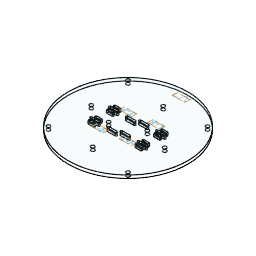
TopPlate_v24 (Autodesk Fusion 360 design; units mm, degrees)
Autodesk Fusion 360 part; units mm, degrees
sketch "Sketch1" plane through (0, 0, 0) normal (0, 0, 1) x (1, 0, 0)
  circle A0 centre (0, 0) radius 59.5
  line L0 (0, -35) -> (0, 35) construction
  circle A1 centre (0, -35) radius 1.75
  circle A2 centre (0, 35) radius 3
  circle A3 centre (0, -35) radius 3
  circle A4 centre (0, 35) radius 6
  circle A5 centre (0, -35) radius 6
  circle A6 centre (0, 35) radius 1.75
  line L1 (0, 0) -> (39.598, 39.598) construction
  line L2 (0, 0) -> (53.8605, 0) construction
  circle A7 centre (39.598, 39.598) radius 1.75
  circle A8 centre (-39.598, 39.598) radius 1.75
  circle A9 centre (-39.598, -39.598) radius 1.75
  circle A10 centre (39.598, -39.598) radius 1.75
  line L3 (-26, 7.75) -> (-1, 7.75) construction
  circle A11 centre (-26, 7.75) radius 1
  circle A12 centre (-1, 7.75) radius 1
  circle A13 centre (-18, 7.75) radius 1
  circle A14 centre (-9, 7.75) radius 1
  line L4 (-26, 8.75) -> (-18, 8.75)
  line L5 (-18, 6.75) -> (-26, 6.75)
  line L6 (-9, 8.75) -> (-1, 8.75)
  line L7 (-1, 6.75) -> (-9, 6.75)
  line L8 (0, 0) -> (-1, 0)
  line L9 (-1, 0) -> (-1, 7.75) construction
  line L10 (26, -8.75) -> (18, -8.75)
  circle A15 centre (26, -7.75) radius 1
  line L11 (18, -6.75) -> (26, -6.75)
  circle A16 centre (18, -7.75) radius 1
  circle A17 centre (9, -7.75) radius 1
  line L12 (9, -8.75) -> (1, -8.75)
  line L13 (1, -6.75) -> (9, -6.75)
  circle A18 centre (1, -7.75) radius 1
  circle A19 centre (9, 10.75) radius 1
  line L14 (0.9757, 9.75) -> (9, 9.75)
  circle A20 centre (1, 10.75) radius 1
  circle A21 centre (18, 10.75) radius 1
  circle A22 centre (26, 10.75) radius 1
  line L15 (9, 11.75) -> (1, 11.75)
  line L16 (0, 0) -> (1, 0)
  line L17 (1, 10.75) -> (26, 10.75) construction
  line L18 (1, 10.75) -> (1, 0) construction
  line L19 (18, 11.75) -> (26, 11.75)
  line L20 (26, 9.75) -> (18, 9.75)
  line L21 (-18, -11.75) -> (-26, -11.75)
  circle A23 centre (-18, -10.75) radius 1
  line L22 (-26, -9.75) -> (-18, -9.75)
  circle A24 centre (-26, -10.75) radius 1
  line L23 (-9, -11.75) -> (-1, -11.75)
  circle A25 centre (-1, -10.75) radius 1
  line L24 (-0.9757, -9.75) -> (-9, -9.75)
  circle A26 centre (-9, -10.75) radius 1
  line L25 (36.6, 0) -> (-36.6, 0) construction
  circle A27 centre (-36.6, 0) radius 1.75
  circle A28 centre (36.6, 0) radius 1.75
  line L26 (13.5, 10.75) -> (13.5, 5.75)
  circle A29 centre (13.5, 5.75) radius 1.75
  circle A30 centre (-13.5, -5.75) radius 1.75
  line L27 (-22, 6.75) -> (-22, 4.5)
  line L28 (-18.9, 3.65) -> (-25.1, 3.65)
  line L29 (-25.1, 3.65) -> (-25.1, 5.35)
  line L30 (-25.1, 5.35) -> (-18.9, 5.35)
  line L31 (-18.9, 5.35) -> (-18.9, 3.65)
  line L32 (-18.9, 3.65) -> (-25.1, 5.35) construction
  line L33 (-25.1, 3.65) -> (-18.9, 5.35) construction
  line L34 (-25.1, 10.15) -> (-18.9, 10.15)
  line L35 (-25.1, 11.85) -> (-25.1, 10.15)
  line L36 (-18.9, 11.85) -> (-25.1, 11.85)
  line L37 (-18.9, 10.15) -> (-18.9, 11.85)
  line L38 (-11.85, -18.9) -> (-11.85, -25.1)
  line L39 (-11.85, -25.1) -> (-10.15, -25.1)
  line L40 (-10.15, -25.1) -> (-10.15, -18.9)
  line L41 (-10.15, -18.9) -> (-11.85, -18.9)
  line L42 (-5.35, -25.1) -> (-5.35, -18.9)
  line L43 (-3.65, -25.1) -> (-5.35, -25.1)
  line L44 (-3.65, -18.9) -> (-3.65, -25.1)
  line L45 (-5.35, -18.9) -> (-3.65, -18.9)
  line L46 (18.9, -11.85) -> (25.1, -11.85)
  line L47 (25.1, -11.85) -> (25.1, -10.15)
  line L48 (25.1, -10.15) -> (18.9, -10.15)
  line L49 (18.9, -10.15) -> (18.9, -11.85)
  line L50 (25.1, -5.35) -> (18.9, -5.35)
  line L51 (25.1, -3.65) -> (25.1, -5.35)
  line L52 (18.9, -3.65) -> (25.1, -3.65)
  line L53 (18.9, -5.35) -> (18.9, -3.65)
  line L54 (11.85, 18.9) -> (11.85, 25.1)
  line L55 (11.85, 25.1) -> (10.15, 25.1)
  line L56 (10.15, 25.1) -> (10.15, 18.9)
  line L57 (10.15, 18.9) -> (11.85, 18.9)
  line L58 (5.35, 25.1) -> (5.35, 18.9)
  line L59 (3.65, 25.1) -> (5.35, 25.1)
  line L60 (3.65, 18.9) -> (3.65, 25.1)
  line L61 (5.35, 18.9) -> (3.65, 18.9)
  line L62 (22, 9.75) -> (22, 7.5)
  line L63 (25.1, 6.65) -> (18.9, 6.65)
  line L64 (18.9, 6.65) -> (18.9, 8.35)
  line L65 (18.9, 8.35) -> (25.1, 8.35)
  line L66 (25.1, 8.35) -> (25.1, 6.65)
  line L67 (25.1, 6.65) -> (18.9, 8.35) construction
  line L68 (18.9, 6.65) -> (25.1, 8.35) construction
  line L69 (18.9, 13.15) -> (25.1, 13.15)
  line L70 (18.9, 14.85) -> (18.9, 13.15)
  line L71 (25.1, 14.85) -> (18.9, 14.85)
  line L72 (25.1, 13.15) -> (25.1, 14.85)
  line L73 (-14.85, 25.1) -> (-14.85, 18.9)
  line L74 (-14.85, 18.9) -> (-13.15, 18.9)
  line L75 (-13.15, 18.9) -> (-13.15, 25.1)
  line L76 (-13.15, 25.1) -> (-14.85, 25.1)
  line L77 (-8.35, 18.9) -> (-8.35, 25.1)
  line L78 (-8.35, 25.1) -> (-6.65, 25.1)
  line L79 (-6.65, 25.1) -> (-6.65, 18.9)
  line L80 (-6.65, 18.9) -> (-8.35, 18.9)
  line L81 (-25.1, -14.85) -> (-18.9, -14.85)
  line L82 (-18.9, -14.85) -> (-18.9, -13.15)
  line L83 (-18.9, -13.15) -> (-25.1, -13.15)
  line L84 (-25.1, -13.15) -> (-25.1, -14.85)
  line L85 (-18.9, -8.35) -> (-25.1, -8.35)
  line L86 (-25.1, -8.35) -> (-25.1, -6.65)
  line L87 (-25.1, -6.65) -> (-18.9, -6.65)
  line L88 (-18.9, -6.65) -> (-18.9, -8.35)
  line L89 (14.85, -25.1) -> (14.85, -18.9)
  line L90 (14.85, -18.9) -> (13.15, -18.9)
  line L91 (13.15, -18.9) -> (13.15, -25.1)
  line L92 (13.15, -25.1) -> (14.85, -25.1)
  line L93 (8.35, -18.9) -> (8.35, -25.1)
  line L94 (8.35, -25.1) -> (6.65, -25.1)
  line L95 (6.65, -25.1) -> (6.65, -18.9)
  line L96 (6.65, -18.9) -> (8.35, -18.9)
  point P0 (-22, 4.5)
  point P1 (22, 7.5)
  dimension "d67" = 119
  dimension "d74" = 3.5
  dimension "d75" = 6
  dimension "d78" = 12
  dimension "d109" = 12
  dimension "d110" = 6
  dimension "d111" = 3.5
  dimension "d112" = 45
  dimension "d113" = 56
  dimension "d114" = 3.5
  dimension "d116" = 360
  dimension "d117" = 25
  dimension "d118" = 2
  dimension "d119" = 2
  dimension "d120" = 2
  dimension "d121" = 2
  dimension "d122" = 8
  dimension "d123" = 8
  dimension "d124" = 1
  dimension "d125" = 7.75
  dimension "d127" = 360
  dimension "d129" = 1
  dimension "d131" = 10.75
  dimension "d132" = 25
  dimension "d133" = 2
  dimension "d134" = 2
  dimension "d135" = 2
  dimension "d136" = 2
  dimension "d137" = 8
  dimension "d138" = 8
  dimension "d140" = 360
  dimension "d141" = 73.2
  dimension "d142" = 3.5
  dimension "d143" = 3.5
  dimension "d144" = 5
  dimension "d145" = 3.5
  dimension "d146" = 2.25
  dimension "d147" = 6.2
  dimension "d148" = 1.7
  dimension "d149" = 2.25
  dimension "d150" = 6.2
  dimension "d151" = 1.7
  constraint coincident A0.centre L1.start
  constraint midpoint L0 A0.centre
  constraint coincident L0.start A1.centre
  constraint coincident L0.end A2.centre
  constraint concentric A1 A3
  constraint concentric A2 A4
  constraint concentric A3 A5
  constraint concentric A2 A6
  constraint horizontal L2
  constraint coincident L1.end A7.centre
  constraint horizontal L3
  constraint coincident L3.start A11.centre
  constraint coincident L3.end A12.centre
  constraint coincident L3 A13.centre
  constraint coincident L3 A14.centre
  constraint coincident A11 L4.start
  constraint coincident A13 L4.end
  constraint coincident A13 L5.start
  constraint coincident A11 L5.end
  constraint coincident A14 L6.start
  constraint coincident A12 L6.end
  constraint coincident A12 L7.start
  constraint coincident A14 L7.end
  constraint tangent A11 L4
  constraint tangent A13 L4
  constraint tangent A13 L5
  constraint tangent A11 L5
  constraint tangent A14 L6
  constraint tangent A14 L7
  constraint tangent A12 L6
  constraint tangent A12 L7
  constraint perpendicular L0 L8
  constraint perpendicular L8 L9
  constraint horizontal L8
  constraint coincident A20.centre L17.start
  constraint coincident A22.centre L17.end
  constraint horizontal L17
  constraint tangent A19 L14
  constraint tangent A19 L15
  constraint tangent A20 L15
  constraint tangent L14 A20
  constraint perpendicular L2 L18
  constraint horizontal L16
  constraint coincident A19.centre L17
  constraint coincident A21.centre L17
  constraint coincident A21 L19.start
  constraint coincident A22 L19.end
  constraint coincident A22 L20.start
  constraint coincident A21 L20.end
  constraint tangent A21 L19
  constraint tangent A22 L19
  constraint tangent A22 L20
  constraint tangent A21 L20
  constraint midpoint A0.centre L25
  constraint perpendicular L9 L25
  constraint coincident L25.end A27.centre
  constraint coincident L25.start A28.centre
  constraint midpoint L17 L26.start
  constraint perpendicular L17 L26
  constraint coincident L26.end A29.centre
  constraint coincident A19 L15.start
  constraint coincident A19 L14.end
  constraint coincident A20 L15.end
  constraint midpoint L5 L27.start
  constraint perpendicular L20 L27
  constraint horizontal L28
  constraint perpendicular L28 L29
  constraint parallel L28 L30
  constraint parallel L29 L31
  constraint coincident L32 P0
  constraint coincident L33 P0
  constraint coincident P0 L27.end
  constraint symmetric L3 L28.start L36.start
  constraint symmetric L3 L28.end L35.start
  constraint symmetric L3 L29.end L34.start
  constraint symmetric L3 L30.end L34.end
  constraint midpoint L20 L62.start
  constraint perpendicular L20 L62
  constraint horizontal L63
  constraint perpendicular L63 L64
  constraint parallel L63 L65
  constraint parallel L64 L66
  constraint coincident L67 P1
  constraint coincident L68 P1
  constraint coincident P1 L62.end
  constraint symmetric L17 L63.start L71.start
  constraint symmetric L17 L63.end L70.start
  constraint symmetric L17 L64.end L69.start
  constraint symmetric L17 L65.end L69.end
  measures "d67" diameter of A0
  measures "d74" diameter of A1
  measures "d75" diameter of A2
  measures "d78" diameter of A4
  measures "d109" diameter of A5
  measures "d110" diameter of A3
  measures "d111" diameter of A6
  measures "d112" angle of L1 L2
  measures "d113" distance of A0.centre L1.end
  measures "d114" diameter of A7
  measures "d117" distance of L3.start L3.end
  measures "d118" diameter of A11
  measures "d119" diameter of A12
  measures "d120" diameter of A13
  measures "d121" diameter of A14
  measures "d122" distance of L3.start A13.centre
  measures "d123" distance of L3.end A14.centre
  measures "d124" distance of A0.centre L8.end
  measures "d125" distance of L8.end L3.end
  measures "d129" distance of A0.centre L16.end
  measures "d131" distance of L16.end A20.centre
  measures "d132" distance of A20.centre A22.centre
  measures "d133" diameter of A20
  measures "d134" diameter of A19
  measures "d135" diameter of A21
  measures "d136" diameter of A22
  measures "d137" horizontal distance of A19.centre A20.centre
  measures "d138" horizontal distance of A21.centre A22.centre
  measures "d141" distance of L25.start L25.end
  measures "d142" diameter of A27
  measures "d143" diameter of A28
  measures "d144" distance of L26.start L26.end
  measures "d145" diameter of A29
  measures "d146" distance of L27.start P0
  measures "d147" distance of L29.end L30.end
  measures "d148" distance of L28.end L29.end
  measures "d149" distance of L62.start P1
  measures "d150" distance of L64.end L65.end
  measures "d151" distance of L63.end L64.end
extrude "Extrude6" add sketch "Sketch1" against normal blind 3 contours A0 | A2 | A3 | A4 | A5 | L38 L39 L40 L41 | L42 L43 L44 L45 | L54 L55 L56 L57 | L58 L59 L60 L61 | L73 L74 L75 L76 | L77 L78 L79 L80 | L89 L90 L91 L92 | L93 L94 L95 L96
sketch "Sketch4" plane through (0, 0, 0) normal (0, 0, 1) x (-1, 0, 0)
  arc A0 (9, -8.75) -> (9, -6.75) centre (9, -7.75) ccw
  line L0 (9, -8.75) -> (1, -8.75)
  arc A1 (1, -6.75) -> (1, -8.75) centre (1, -7.75) ccw
  line L1 (1, -6.75) -> (9, -6.75)
  line L2 (-25.1, -14.85) -> (-25.1, -13.15)
  line L3 (-25.1, -13.15) -> (-18.9, -13.15)
  line L4 (-18.9, -13.15) -> (-18.9, -14.85)
  line L5 (-18.9, -14.85) -> (-25.1, -14.85)
  arc A2 (9, 9.75) -> (9, 11.75) centre (9, 10.75) ccw
  line L6 (9, 9.75) -> (1, 9.75)
  arc A3 (1, 11.75) -> (1, 9.75) centre (1, 10.75) ccw
  line L7 (1, 11.75) -> (9, 11.75)
  circle A4 centre (-13.5, -5.75) radius 1.75
  line L8 (-25.1, 5.35) -> (-18.9, 5.35)
  line L9 (-18.9, 5.35) -> (-18.9, 3.65)
  line L10 (-18.9, 3.65) -> (-25.1, 3.65)
  line L11 (-25.1, 3.65) -> (-25.1, 5.35)
  circle A5 centre (0, -35) radius 1.75
  line L12 (-18.9, -8.35) -> (-25.1, -8.35)
  line L13 (-25.1, -8.35) -> (-25.1, -6.65)
  line L14 (-25.1, -6.65) -> (-18.9, -6.65)
  line L15 (-18.9, -6.65) -> (-18.9, -8.35)
  line L16 (18.9, -11.85) -> (18.9, -10.15)
  line L17 (18.9, -10.15) -> (25.1, -10.15)
  line L18 (25.1, -10.15) -> (25.1, -11.85)
  line L19 (25.1, -11.85) -> (18.9, -11.85)
  line L20 (25.1, -5.35) -> (18.9, -5.35)
  line L21 (18.9, -5.35) -> (18.9, -3.65)
  line L22 (18.9, -3.65) -> (25.1, -3.65)
  line L23 (25.1, -3.65) -> (25.1, -5.35)
  circle A6 centre (0, 0) radius 59.5
  circle A7 centre (-36.6, 0) radius 1.75
  line L24 (-1, -11.75) -> (-9, -11.75)
  arc A8 (-9, -9.75) -> (-9, -11.75) centre (-9, -10.75) ccw
  line L25 (-9, -9.75) -> (-1, -9.75)
  arc A9 (-1, -11.75) -> (-1, -9.75) centre (-1, -10.75) ccw
  arc A10 (-18, -11.75) -> (-18, -9.75) centre (-18, -10.75) ccw
  line L26 (-18, -11.75) -> (-26, -11.75)
  arc A11 (-26, -9.75) -> (-26, -11.75) centre (-26, -10.75) ccw
  line L27 (-26, -9.75) -> (-18, -9.75)
  circle A12 centre (-39.598, -39.598) radius 1.75
  line L28 (25.1, 6.65) -> (18.9, 6.65)
  line L29 (18.9, 6.65) -> (18.9, 8.35)
  line L30 (18.9, 8.35) -> (25.1, 8.35)
  line L31 (25.1, 8.35) -> (25.1, 6.65)
  arc A13 (-9, 8.75) -> (-9, 6.75) centre (-9, 7.75) ccw
  line L32 (-9, 8.75) -> (-1, 8.75)
  arc A14 (-1, 6.75) -> (-1, 8.75) centre (-1, 7.75) ccw
  line L33 (-1, 6.75) -> (-9, 6.75)
  arc A15 (-26, 8.75) -> (-26, 6.75) centre (-26, 7.75) ccw
  line L34 (-26, 8.75) -> (-18, 8.75)
  arc A16 (-18, 6.75) -> (-18, 8.75) centre (-18, 7.75) ccw
  line L35 (-18, 6.75) -> (-26, 6.75)
  circle A17 centre (39.598, -39.598) radius 1.75
  circle A18 centre (13.5, 5.75) radius 1.75
  arc A19 (18, 11.75) -> (18, 9.75) centre (18, 10.75) ccw
  line L36 (18, 11.75) -> (26, 11.75)
  arc A20 (26, 9.75) -> (26, 11.75) centre (26, 10.75) ccw
  line L37 (26, 9.75) -> (18, 9.75)
  circle A21 centre (36.6, 0) radius 1.75
  line L38 (25.1, 14.85) -> (25.1, 13.15)
  line L39 (25.1, 13.15) -> (18.9, 13.15)
  line L40 (18.9, 13.15) -> (18.9, 14.85)
  line L41 (18.9, 14.85) -> (25.1, 14.85)
  circle A22 centre (0, 35) radius 1.75
  line L42 (-18.9, 11.85) -> (-18.9, 10.15)
  line L43 (-18.9, 10.15) -> (-25.1, 10.15)
  line L44 (-25.1, 10.15) -> (-25.1, 11.85)
  line L45 (-25.1, 11.85) -> (-18.9, 11.85)
  circle A23 centre (39.598, 39.598) radius 1.75
  circle A24 centre (-39.598, 39.598) radius 1.75
  arc A25 (26, -8.75) -> (26, -6.75) centre (26, -7.75) ccw
  line L46 (26, -8.75) -> (18, -8.75)
  arc A26 (18, -6.75) -> (18, -8.75) centre (18, -7.75) ccw
  line L47 (18, -6.75) -> (26, -6.75)
  line L48 (-7.7229, -53.8276) -> (4.2771, -53.8276) construction
  line L49 (4.2771, -53.8276) -> (4.2771, -48.8276) construction
  line L50 (4.2771, -48.8276) -> (-7.7229, -48.8276) construction
  line L51 (-7.7229, -48.8276) -> (-7.7229, -53.8276) construction
  line L52 (6.481, -14.9209) -> (18.481, -14.9209) construction
  line L53 (18.481, -14.9209) -> (18.481, -9.9209) construction
  line L54 (18.481, -9.9209) -> (6.481, -9.9209) construction
  line L55 (6.481, -9.9209) -> (6.481, -14.9209) construction
  line L56 (18.4787, 18.0791) -> (6.4787, 18.0791) construction
  line L57 (6.4787, 18.0791) -> (6.4787, 13.0791) construction
  line L58 (6.4787, 13.0791) -> (18.4787, 13.0791) construction
  line L59 (18.4787, 13.0791) -> (18.4787, 18.0791) construction
  line L60 (-18.5149, -17.9209) -> (-6.5149, -17.9209) construction
  line L61 (-6.5149, -17.9209) -> (-6.5149, -12.9209) construction
  line L62 (-6.5149, -12.9209) -> (-18.5149, -12.9209) construction
  line L63 (-18.5149, -12.9209) -> (-18.5149, -17.9209) construction
  line L64 (-6.5172, 15.0791) -> (-18.5172, 15.0791) construction
  line L65 (-18.5172, 15.0791) -> (-18.5172, 10.0791) construction
  line L66 (-18.5172, 10.0791) -> (-6.5172, 10.0791) construction
  line L67 (-6.5172, 10.0791) -> (-6.5172, 15.0791) construction
  dimension "d154" = 8
  dimension "d155" = 0
  dimension "d156" = 6
  dimension "d158" = 6
  dimension "d160" = 6
  dimension "d162" = 6
equation "d146 = 1.5 mm + 0.75 mm"
equation "d149 = 1.5 mm + 0.75 mm"
equation "d155 = 'V2'"
equation "d157 = 'T-F'"
equation "d159 = 'L-B'"
equation "d161 = 'L-B'"
equation "d163 = 'T-F'"
